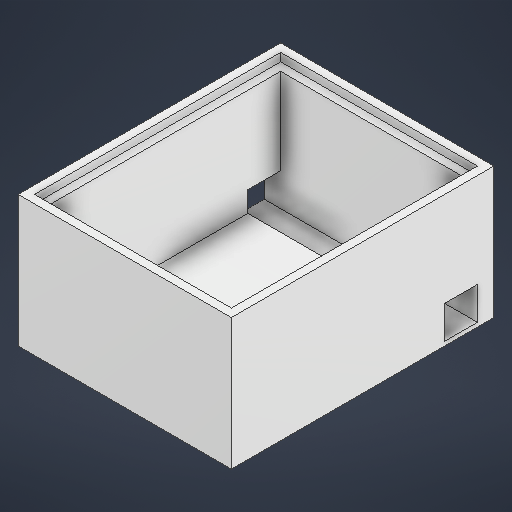
# Autodesk Inventor part: OGRobotBase
Saved by Autodesk Inventor 2027 (Build 310192060, 192F)
## iProperties
Created: 2026-07-04
Part Number: OGRobotBase
Material: ABS Plastic
Document SubType Name: Modeling
Designer: machnach0
Density: 1.06 g/cm^3
Appearance: Smooth - White
Author: machnach0
Autodesk Inventor part; units mm, degrees
ref_plane "YZ Plane" through (0, 0, 0) normal (1, 0, 0) x (0, 1, 0)
ref_plane "XZ Plane" through (0, 0, 0) normal (0, 1, 0) x (-1, 0, 0)
ref_plane "XY Plane" through (0, 0, 0) normal (0, 0, 1) x (1, 0, 0)
sketch "Sketch1" plane through (0, 0, 0) normal (0, 1, 0) x (-1, 0, 0)
  line L0 (0, 0) -> (165.1, 0)
  line L1 (165.1, 0) -> (165.1, -203.2)
  line L2 (165.1, -203.2) -> (0, -203.2)
  line L3 (0, -203.2) -> (0, 0)
  line L4 (158.75, -196.85) -> (158.75, -6.35)
  line L5 (158.75, -6.35) -> (6.35, -6.35)
  line L6 (6.35, -6.35) -> (6.35, -196.85)
  line L7 (6.35, -196.85) -> (158.75, -196.85)
  line L8 (152.4, -190.5) -> (152.4, -12.7)
  line L9 (152.4, -12.7) -> (12.7, -12.7)
  line L10 (12.7, -12.7) -> (12.7, -190.5)
  line L11 (12.7, -190.5) -> (152.4, -190.5)
  dimension "d0" = 203.2
  dimension "d1" = 165.1
  dimension "d2" = 6.35
  dimension "d3" = 12.7
  constraints: 24 end point, 6 parallel, 3 perpendicular, 1 horizontal, 6 other
  measures "d0" distance of L0.end L1.end
  measures "d1" distance of L1.end L2.end
  measures "d2" distance between parallel lines of L2 L7
  measures "d3" distance between parallel lines of L2 L11
extrude "Extrusion1" add sketch "Sketch1" along normal blind 12.7 contours L0 L1 L2 L3 | L7 L6 L5 L4 | L11 L10 L9 L8
extrude "Extrusion2" add sketch "Sketch1" along normal blind 101.6 contours L0 L1 L2 L3
extrude "Extrusion3" add sketch "Sketch1" along normal blind 95.25 contours L7 L6 L5 L4
sketch "Sketch2" plane through (-165.1, 0, -203.2) normal (-1, 0, 0) x (0, 0, 1)
  line L0 (12.7, 12.7) -> (190.5, 12.7) projected
  line L1 (12.7, 28.575) -> (38.1, 28.575)
  line L2 (38.1, 28.575) -> (38.1, 3.175)
  line L3 (38.1, 3.175) -> (12.7, 3.175)
  line L4 (12.7, 3.175) -> (12.7, 28.575)
  line L5 (0, 0) -> (203.2, 0) projected
  dimension "d10" = 3.175
  dimension "d11" = 25.4
  dimension "d12" = 25.4
  constraints: 8 end point, 2 parallel, 1 horizontal, 1 perpendicular, 1 point on line
  measures "d10" distance between parallel lines of L5 L3
  measures "d11" distance between parallel lines of L3 L1
  measures "d12" distance between parallel lines of L2 L4
extrude "Extrusion4" cut sketch "Sketch2" against normal through all
body "Solid1"
